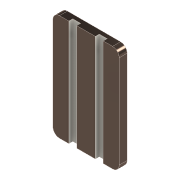
# Autodesk Inventor part: Plate
Saved by Autodesk Inventor 2022.2 (Build 262287010, 287A)
## iProperties
Created: 2022-12-29
Part Number: Plate
Material: Steel
Document SubType Name: Modeling
Designer: User
Mass: 164.781 g
Surface Area: 103.536 cm^2
Volume: 20.9912 cm^3
Density: 7.85 g/cm^3
Appearance: Gunmetal - Antique Polished
Author: User
Autodesk Inventor part; units mm, degrees
ref_plane "YZ Plane" through (0, 0, 0) normal (1, 0, 0) x (0, 1, 0)
ref_plane "XZ Plane" through (0, 0, 0) normal (0, 1, 0) x (-1, 0, 0)
ref_plane "XY Plane" through (0, 0, 0) normal (0, 0, 1) x (1, 0, 0)
sketch "Sketch1" plane through (0, 0, 0) normal (0, 0, 1) x (1, 0, 0)
  line L0 (-25, -40) -> (25, -40)
  line L1 (25, -40) -> (25, 40)
  line L2 (25, 40) -> (-25, 40)
  line L3 (-25, 40) -> (-25, -40)
  line L4 (-25, -40) -> (25, 40) construction
  line L5 (25, -40) -> (-25, 40) construction
  point P0 (0, 0)
  dimension "d0" = 50
  dimension "d1" = 80
  constraints: 12 end point, 2 midpoint, 2 parallel, 1 horizontal, 1 perpendicular
  measures "d0" distance of L2.end L1.end
  measures "d1" distance of L1.end L0.end
extrude "Extrusion1" add sketch "Sketch1" along normal blind 6
sketch "Sketch2" plane through (-25, -40, 0) normal (0, -1, 0) x (1, 0, 0)
  line L0 (0, 6) -> (50, 6) projected
  line L1 (12, 6) -> (18, 6)
  line L2 (18, 6) -> (18, 3)
  line L3 (18, 3) -> (12, 3)
  line L4 (12, 3) -> (12, 6)
  line L5 (32, 6) -> (38, 6)
  line L6 (38, 6) -> (38, 3)
  line L7 (38, 3) -> (32, 3)
  line L8 (32, 3) -> (32, 6)
  line L9 (25, -1.2) -> (25, 7.2) construction
  line L10 (0, 0) -> (50, 0) construction
  line L11 (50, 0) -> (50, 6) construction
  line L12 (0, 6) -> (50, 6) construction
  line L13 (0, 0) -> (0, 6) construction
  point P0 (25, 0)
  point P1 (32, 4.5)
  point P2 (18, 4.5)
  dimension "d4" = 14
  dimension "d5" = 6
  dimension "d7" = 3
  constraints: 16 end point, 4 parallel, 2 horizontal, 2 midpoint, 2 perpendicular, 2 point on line, 1 collinear, 2 other
  measures "d4" distance of point (32, 4.5) point (18, 4.5)
  measures "d5" distance from line of L2.end L4
  measures "d7" distance between parallel lines of L3 L1
extrude "Extrusion2" cut sketch "Sketch2" against normal through all
fillet "Fillet1" radius 5 4 edges at (-25, 40, 3) (-25, -40, 3) (25, -40, 3) (25, 40, 3)
body "Solid1"
